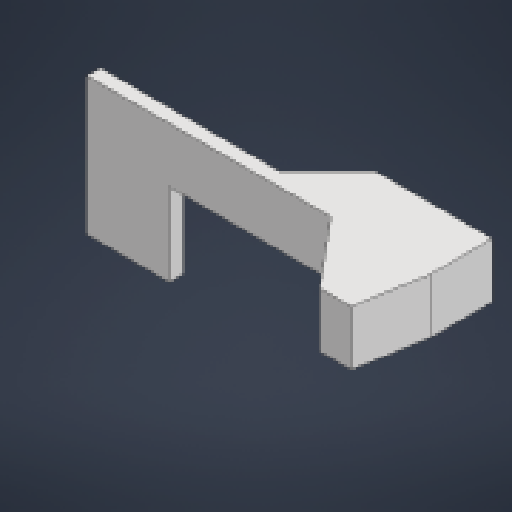
# Autodesk Inventor part: botton
Saved by Autodesk Inventor 2026.2 (Build 302298010, 298A)
## iProperties
Created: 2026-04-05
Part Number: botton
Material: 一般
Document SubType Name: Modeling
Designer: gavin
Density: 1 g/cm^3
Appearance: 預設
Author: gavin
## iProperties of the stored document botton_3D 列印.ipt
Created: 2026-04-05
Part Number: botton_3D 列印
Material: 一般
Document SubType Name: Modeling
Designer: gavin
Density: 1 g/cm^3
Appearance: 預設
Author: gavin
Autodesk Inventor part; units mm, degrees
ref_plane "YZ Plane" through (0, 0, 0) normal (1, 0, 0) x (0, 1, 0)
ref_plane "XZ Plane" through (0, 0, 0) normal (0, 1, 0) x (-1, 0, 0)
ref_plane "XY Plane" through (0, 0, 0) normal (0, 0, 1) x (1, 0, 0)
sketch "草圖1" plane through (0, 0, 0) normal (0, 0, 1) x (1, 0, 0)
  line L0 (0, 0) -> (25, 0)
  line L1 (25, 0) -> (25, -10)
  line L2 (25, -10) -> (0, -10)
  line L3 (0, -10) -> (0, 0)
  line L4 (25, 0) -> (7, 0)
  line L5 (7, 0) -> (7, -4)
  line L6 (7, -4) -> (25, -4)
  line L7 (25, -4) -> (25, 0)
  line L8 (26, -5) -> (6, -5)
  line L9 (6, -5) -> (6, 1)
  line L10 (6, 1) -> (26, 1)
  line L11 (26, 1) -> (26, -5)
  line L12 (7, -4) -> (6, -4)
  line L13 (6, -5) -> (6, -10)
  point P0 (25, -5)
  dimension "d0" = 25
  dimension "d1" = 10
  dimension "d2" = 18
  dimension "d3" = 4
  dimension "d4" = 1
  constraints: 28 end point, 6 parallel, 5 perpendicular, 2 horizontal, 2 point on line, 3 other
  measures "d0" distance of L1.end L2.end
  measures "d1" distance of L0.end L1.end
  measures "d2" distance of L6.end L5.end
  measures "d3" distance of L5.end L4.end
  measures "d4" distance between parallel lines of L6 L8
extrude "擠出1" add sketch "草圖1" along normal blind 1 contours L5 L12 L9 L0 | L0 L1 L6 L5 | L9 L13 L2 L3 L0
sketch "草圖2" plane through (0, 0, 0) normal (0, 1, 0) x (1, 0, 0)
  line L0 (25, -1) -> (0, -1) projected
  line L1 (25, -1) -> (24.136, -5.9)
  line L2 (24.136, -5.9) -> (21.864, -5.9)
  line L3 (21.864, -5.9) -> (17.7524, -1)
  point P0 (0, 0)
  point P1 (23, -5.9)
  dimension "d7" = 4.9
  dimension "d8" = 2
  dimension "d9" = 80
  dimension "d10" = 50
  constraints: 6 end point, 1 horizontal, 1 midpoint, 1 point on line
  measures "d7" distance between parallel lines of L2 L0
  measures "d8" horizontal distance of L0.start point (23, -5.9)
  measures "d9" angle of L0 L1
  measures "d10" angle of L0 L3
extrude "擠出2" add sketch "草圖2" against normal up to surface (4 mm away)
sketch "草圖3" plane through (0, 0, 0) normal (0, 1, 0) x (1, 0, 0)
  line L0 (25, 0) -> (0, 0) projected
  line L1 (0, 0) -> (0, -1) projected
  line L2 (17.7524, -1) -> (0, -1) projected
  line L3 (17.7524, -1) -> (21.864, -5.9) projected
  line L4 (21.864, -5.9) -> (24.136, -5.9) projected
  line L5 (24.136, -5.9) -> (25, -1) projected
  line L6 (25, 0) -> (25, -1) projected
  line L7 (25, 0) -> (25, 3.5)
  line L8 (25, 3.5) -> (16.5, 3.5)
  line L9 (16.5, 3.5) -> (13, 0)
  dimension "d13" = 12
  dimension "d14" = 45
  dimension "d15" = 3.5
  constraints: 6 end point, 1 perpendicular, 1 point on line, 1 vertical
  measures "d13" distance from line of L9.end L7
  measures "d14" angle of L0 L9
  measures "d15" distance between parallel lines of L0 L8
extrude "擠出3" add sketch "草圖3" against normal up to surface (4 mm away) contours L0 L9 L8 L7
